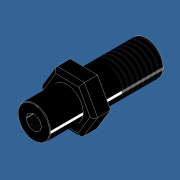
# Autodesk Inventor part: Double Sided Bolt
Saved by Autodesk Inventor 2018 (Build 220112000, 112)
## iProperties
Created: 2018-02-28
Part Number: Double Sided Bolt
Material: Stainless Steel
Document SubType Name: Modeling
Designer: 232963
Density: 8 g/cm^3
Appearance: Chrome - Polished
Author: 232963
Autodesk Inventor part; units mm, degrees
ref_plane "YZ Plane" through (0, 0, 0) normal (1, 0, 0) x (0, 1, 0)
ref_plane "XZ Plane" through (0, 0, 0) normal (0, 1, 0) x (-1, 0, 0)
ref_plane "XY Plane" through (0, 0, 0) normal (0, 0, 1) x (1, 0, 0)
sketch "Sketch1" plane through (0, 0, 0) normal (0, 0, 1) x (1, 0, 0)
  line L0 (6.4577, 10.7072) -> (12.5016, -0.2389)
  line L1 (12.5016, -0.2389) -> (6.0439, -10.9461)
  line L2 (6.0439, -10.9461) -> (-6.4577, -10.7072)
  line L3 (-6.4577, -10.7072) -> (-12.5016, 0.2389)
  line L4 (-12.5016, 0.2389) -> (-6.0439, 10.9461)
  line L5 (-6.0439, 10.9461) -> (6.4577, 10.7072)
  point P0 (0, 0)
  point P1 (0, 0)
  dimension "d0" = 25.0031
  constraints: 12 end point, 1 coincident, 13 other
  measures "d0" horizontal distance of L0.end L3.end
extrude "Extrusion1" add sketch "Sketch1" along normal mid plane 7.874
sketch "Sketch2" plane through (0, 0, 3.937) normal (0, 0, 1) x (1, 0, 0)
  circle A0 centre (0, 0) radius 7.4676
  dimension "d3" = 14.9352
  constraints: 1 centre point, 1 coincident
  measures "d3" diameter of A0
extrude "Extrusion2" add sketch "Sketch2" along normal blind 15.24
fillet "Fillet1" radius 0.254 1 edges at (-7.4676, 0, 19.177)
sketch "Sketch3" plane through (0, 0, 19.177) normal (0, 0, 1) x (1, 0, 0)
  point P0 (0, 0)
  point P1 (0, 0)
  constraints: 1 coincident
hole "Hole1" at (0, 0, 19.177) at (0, 0, 19.177) direction (0, 0, -1) diameter 6.7469 depth 15.24
sketch "Sketch4" plane through (0, 0, -3.937) normal (0, 0, -1) x (-1, 0, 0)
  circle A0 centre (0, 0) radius 7.8105
  dimension "d15" = 15.621
  constraints: 1 centre point, 1 coincident
  measures "d15" diameter of A0
extrude "Extrusion3" add sketch "Sketch4" along normal blind 28.575
thread "Thread1" size "5/8-11 UNC" class "2A" standard "ANSI Unified Screw Threads" length 19.05
thread "Thread2" size "10-24 UNC" class "2B" standard "ANSI Unified Screw Threads" length 25.4
fillet "Fillet2" radius 1.5875 6 edges at (9.4796, 5.2342, 3.937) (0.2069, 10.8267, 3.937) (9.2727, -5.5925, 3.937) (-0.2069, -10.8267, 3.937) (-9.4796, -5.2342, 3.937) (-9.2727, 5.5925, 3.937)
fillet "Fillet3" radius 0.3175 6 edges at (-0.2069, -10.8267, -3.937) (9.2727, -5.5925, -3.937) (9.4796, 5.2342, -3.937) (0.2069, 10.8267, -3.937) (-9.2727, 5.5925, -3.937) (-9.4796, -5.2342, -3.937)
body "Solid1"
